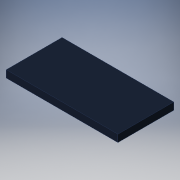
# Autodesk Inventor part: Phone
Saved by Autodesk Inventor 2019 (Build 230136000, 136)
## iProperties
Created: 2019-10-11
Part Number: Phone
Material: Generic
Document SubType Name: Modeling
Designer: james
Density: 1 g/cm^3
Appearance: Default(1)
Author: james
Autodesk Inventor part; units mm, degrees
ref_plane "YZ Plane" through (0, 0, 0) normal (1, 0, 0) x (0, 1, 0)
ref_plane "XZ Plane" through (0, 0, 0) normal (0, 1, 0) x (-1, 0, 0)
ref_plane "XY Plane" through (0, 0, 0) normal (0, 0, 1) x (1, 0, 0)
sketch "Sketch1" plane through (0, 0, 0) normal (0, 1, 0) x (-1, 0, 0)
  line L0 (46.1101, 42.2596) -> (-98.6699, 42.2596)
  line L1 (-98.6699, 42.2596) -> (-98.6699, -30.1304)
  line L2 (-98.6699, -30.1304) -> (46.1101, -30.1304)
  line L3 (46.1101, -30.1304) -> (46.1101, 42.2596)
  point P0 (0, 0)
  dimension "d2" = 72.39
  dimension "d3" = 144.78
  constraints: 8 end point, 2 parallel, 1 horizontal, 1 perpendicular
  measures "d2" distance of L2.end L0.start
  measures "d3" distance of L0.start L0.end
extrude "Extrusion1" add sketch "Sketch1" along normal blind 9.398
body "Solid1"
